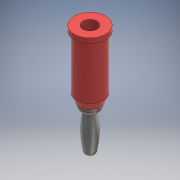
# Autodesk Inventor part: 05-0007
Saved by Autodesk Inventor 2018 (Build 220112000, 112)
## iProperties
Created: 2019-09-30
Part Number: 05-0007
Material: ABS Plastic
Document SubType Name: Modeling
Designer: Bradley
Density: 1.06 g/cm^3
Appearance: Smooth - Red
Author: Bradley
Autodesk Inventor part; units mm, degrees
ref_plane "YZ Plane" through (0, 0, 0) normal (1, 0, 0) x (0, 1, 0)
ref_plane "XZ Plane" through (0, 0, 0) normal (0, 1, 0) x (-1, 0, 0)
ref_plane "XY Plane" through (0, 0, 0) normal (0, 0, 1) x (1, 0, 0)
sketch "Sketch1" plane through (0, 0, 0) normal (0, 1, 0) x (-1, 0, 0)
  line L0 (0, -13.3) -> (0, 13.3)
  line L1 (0, 13.3) -> (-2.5, 13.3)
  line L2 (-2.5, 13.3) -> (-2.5, 26.3)
  line L3 (-2.5, 26.3) -> (-5.55, 26.3)
  line L4 (-5.55, 26.3) -> (-5.55, 24.6)
  line L5 (-5.55, 24.6) -> (-4.75, 24.6)
  line L6 (-4.75, 24.6) -> (-4.75, 5.7)
  line L7 (-4.75, 5.7) -> (-3.7, 3.2)
  line L8 (-3.7, 3.2) -> (-3.2, 3.2)
  line L9 (-3.2, 3.2) -> (-3.2, 1.9)
  line L10 (-1.8, 0.6) -> (-1.8, 0.5)
  arc A0 (-1.8, 0.5) -> (-1.8, -11.8195) centre (29.519, -5.6598) ccw
  arc A1 (-1.8, -11.8195) -> (0, -13.3) centre (0, -11.4655) ccw
  line L11 (-1.8, 0.6) -> (-2.4, 0.6)
  arc A2 (-3.2, 1.9) -> (-2.4, 0.6) centre (-1.7438, 1.9) ccw
  line L12 (-2.4, -5.6598) -> (0, -5.6598) construction
  point P0 (0, 0)
  point P1 (0, 0)
  dimension "d0" = 11.1
  dimension "d1" = 5
  dimension "d2" = 1.7
  dimension "d3" = 23.1
  dimension "d4" = 20.6
  dimension "d5" = 0.1
  dimension "d6" = 1.3
  dimension "d7" = 2.6
  dimension "d8" = 3.6
  dimension "d9" = 6.4
  dimension "d10" = 4.8
  dimension "d11" = 39.6
  dimension "d12" = 13
  dimension "d13" = 9.5
  dimension "d14" = 7.4
  dimension "d15" = 4.8
  constraints: 26 end point, 8 perpendicular, 7 point on circle, 3 centre point, 2 parallel, 2 point on line, 2 tangent, 1 coincident, 1 horizontal, 1 line through centre, 1 midpoint, 1 vertical
  measures "d0" diameter of L4 L0
  measures "d1" diameter of L2 L0
  measures "d2" distance of L3.end L4.end
  measures "d3" distance between parallel lines of L3 L8
  measures "d4" distance from line of L6.end L3
  measures "d5" distance of L10.start L10.end
  measures "d6" distance of L8.end L9.end
  measures "d7" distance from line of L10.start L8
  measures "d8" diameter of L10 L0
  measures "d9" diameter of L9 L0
  measures "d10" diameter of L11.end L0
  measures "d11" distance from line of L3 L0.start
  measures "d12" distance of L1.end L2.end
  measures "d13" diameter of L6 L0
  measures "d14" diameter of L7.end L0
  measures "d15" diameter of L12.start L0
revolve "Revolution1" add sketch "Sketch1" angle 360 about axis through (0, 0, -13.3) along (0, 0, 1)
body "Solid1"
